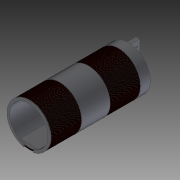
# Autodesk Inventor part: 3113_Rx Coil_V1
Saved by Autodesk Inventor 2020 (Build 240168000, 168)
## iProperties
Created: 2017-07-27
Part Number: 3113_Rx Coil_V1
Material: Acetal Resin, White
Document SubType Name: Modeling
Designer: RFLab
Density: 1.425 g/cm^3
Appearance: Smooth - White
Mass: 82.1964 g
Surface Area: 486.741 cm^2
Volume: 57.6817 cm^3
Author: RFLab
Autodesk Inventor part; units mm, degrees
ref_plane "XZ Plane" through (0, 0, 0) normal (0, 1, 0) x (-1, 0, 0)
ref_plane "XY Plane" through (0, 0, 0) normal (0, 0, 1) x (1, 0, 0)
sketch "Sketch1" plane through (0, 0, 0) normal (1, 0, 0) x (0, 1, 0)
  line L0 (0, 0) -> (0, -63.2887) construction
  line L1 (25, 58.6865) -> (25, -71.3865)
  line L2 (25, -71.3865) -> (28.75, -71.3865)
  line L3 (28.75, -71.3865) -> (28.75, -58.6865)
  line L4 (28.75, -58.6865) -> (26.2, -58.6865)
  line L5 (26.2, -58.6865) -> (26.2, -18.6865)
  line L6 (26.2, -18.6865) -> (28.75, -18.6865)
  line L7 (28.75, -18.6865) -> (28.75, 18.6865)
  line L8 (28.75, 18.6865) -> (26.2, 18.6865)
  line L9 (26.2, 18.6865) -> (26.2, 58.6865)
  line L10 (28.75, 58.6865) -> (25, 58.6865)
  line L11 (26.2, 58.6865) -> (26.2, 58.6865)
  point P0 (28.75, 0)
  dimension "d35" = 25
  dimension "d43" = 12.7
  dimension "d61" = 117.373
  dimension "d62" = 40
  dimension "d63" = 40
  dimension "d64" = 37.373
  dimension "d125" = 1.2
  dimension "d127" = 28.75
  dimension "d128" = 2.55
  constraints: 24 end point, 6 perpendicular, 6 point on line, 3 vertical, 1 collinear, 1 horizontal alignment, 1 midpoint
  measures "d35" distance between parallel lines of L0 L1
  measures "d43" distance of L2.end L3.end
  measures "d61" distance between parallel lines of L4 L10
  measures "d62" distance of L8.end L9.end
  measures "d63" distance of L4.end L5.end
  measures "d64" distance of L6.end L7.end
  measures "d125" distance between parallel lines of L1 L5
  measures "d127" distance between parallel lines of L7 L0
  measures "d128" distance between parallel lines of L5 L3
revolve "Revolution1" add sketch "Sketch1" angle 360 about axis through (0, 0, 0) along (0, 0, -1)
sketch "Sketch2" plane through (0, 0, -71.3865) normal (0, 0, -1) x (-1, 0, 0)
  line L0 (-16.1894, -19.05) -> (-11.1252, -19.05)
  line L1 (-11.1252, -19.05) -> (-11.1252, -23.8252)
  line L2 (-11.1252, -23.8252) -> (-6.35, -23.8252)
  line L3 (-6.35, -23.8252) -> (-6.35, -19.05)
  line L4 (-6.35, -19.05) -> (6.35, -19.05)
  line L5 (6.35, -19.05) -> (6.35, -23.8252)
  line L6 (6.35, -23.8252) -> (11.1252, -23.8252)
  line L7 (11.1252, -23.8252) -> (11.1252, -19.05)
  line L8 (11.1252, -19.05) -> (16.1894, -19.05)
  circle A0 centre (0, 0) radius 25 projected
  arc A1 (-16.1894, -19.05) -> (16.1894, -19.05) centre (0, 0) ccw
  point P0 (0, -19.05)
  dimension "d11" = 19.05
  dimension "d12" = 4.7752
  dimension "d14" = 12.7
  constraints: 18 end point, 6 point on line, 5 perpendicular, 2 equal length, 2 point on circle, 1 centre point, 1 coincident, 1 horizontal, 1 midpoint, 1 vertical alignment, 2 other
  measures "d11" distance from line of L4 point (0, 0)
  measures "d12" distance of L2.end L3.end
  measures "d14" distance of L3.end L4.end
extrude "Extrusion1" [suppressed]
sketch "Sketch4" plane through (0, 0, 0) normal (1, 0, 0) x (0, 1, 0)
  circle A0 centre (26.7715, -19.258) radius 0.5715
  line L0 (-28.75, -18.6865) -> (28.75, -18.6865) projected
  line L1 (26.2, -18.6865) -> (26.2, -58.6865) projected
  point P0 (0, 0)
  point P1 (26.2, -176.784)
  dimension "d22" = 1.143
  constraints: 2 point on line, 1 centre point, 1 tangent, 1 vertical alignment, 3 other
  measures "d22" diameter of A0
sketch "Sketch10" plane through (0, 0, 58.6865) normal (0, 0, 1) x (1, 0, 0)
  circle A0 centre (0, 0) radius 25 projected
  line L0 (-12.193, -21.825) -> (12.193, -21.825)
  line L1 (0, -21.825) -> (0, -25)
  dimension "d45" = 3.175
  constraints: 4 end point, 3 point on circle, 1 horizontal, 1 midpoint, 1 vertical
  measures "d45" distance of L1.start L1.end
extrude "Extrusion5" add sketch "Sketch10" against normal up to surface (130.073 mm away) contours L0 L1 A0 | A0 L1 L0
sketch "Sketch11" plane through (0, 0, 58.6865) normal (0, 0, 1) x (1, 0, 0)
  arc A0 (12.193, -21.825) -> (-12.193, -21.825) centre (0, 0) ccw projected
  line L0 (12.193, -21.825) -> (-12.2967, -21.825)
  line L1 (-12.2967, -21.825) -> (-12.2967, -41.275)
  line L2 (-12.2967, -41.275) -> (12.193, -41.275)
  line L3 (12.193, -41.275) -> (12.193, -21.825)
  line L4 (-6.35, -41.275) -> (6.35, -41.275)
  line L5 (6.35, -41.275) -> (6.35, -21.825)
  line L6 (6.35, -21.825) -> (-6.35, -21.825)
  line L7 (-6.35, -21.825) -> (-6.35, -41.275)
  arc A1 (0, 28.75) -> (0, 28.75) centre (0, 0) ccw projected
  point P0 (0, -41.275)
  point P1 (0, 28.75)
  dimension "d48" = 41.275
  dimension "d49" = 12.7
  constraints: 16 end point, 4 parallel, 2 horizontal, 2 perpendicular, 2 point on line, 1 midpoint, 1 point on circle, 1 vertical alignment
  measures "d48" distance from line of A0.centre L2
  measures "d49" distance between parallel lines of L5 L7
extrude "Extrusion6" add sketch "Sketch11" along normal blind 14 contours L5 A1 L7 L0 | L5 L2 L7 A1
sketch "Sketch12" plane through (0, 0, 72.6865) normal (0, 0, 1) x (1, 0, 0)
  line L0 (6.35, -21.825) -> (-6.35, -21.825) projected
  line L1 (0, -21.825) -> (0, -31.496)
  circle A0 centre (0, -31.496) radius 2.54
  point P0 (0, 0)
  dimension "d52" = 9.671
  dimension "d53" = 5.08
  constraints: 2 coincident, 2 end point, 1 centre point, 1 midpoint, 1 vertical
  measures "d52" distance of L1.start L1.end
  measures "d53" diameter of A0
extrude "Extrusion7" cut sketch "Sketch12" against normal blind 9.525
sketch "Sketch13" plane through (0, 0, 58.6865) normal (0, 0, -1) x (-1, 0, 0)
  arc A0 (-6.35, -27.8605) -> (6.35, -27.8605) centre (0, 0) ccw projected
  line L0 (-6.35, -41.275) -> (-6.35, -25.4188) projected
  line L1 (6.35, -41.275) -> (-6.35, -41.275) projected
  line L2 (6.35, -25.4188) -> (6.35, -41.275) projected
extrude "Extrusion8" cut sketch "Sketch13" against normal blind 8
sketch "Sketch20" plane through (0, 0, 58.6865) normal (0, 0, 1) x (1, 0, 0)
  circle A0 centre (0, 0) radius 28.58
  circle A1 centre (0, 0) radius 25
  dimension "d110" = 57.16
  dimension "d120" = 50
  constraints: 2 centre point, 2 coincident
  measures "d110" diameter of A0
  measures "d120" diameter of A1
extrude "Extrusion14" add sketch "Sketch20" along normal blind 1
ref_plane "Work Plane4" through (-30, 0, 0) normal (1, 0, 0) x (0, 1, 0)
sketch "Sketch29" plane through (-30, 0, 0) normal (1, 0, 0) x (0, 1, 0)
  line L0 (-26.2, 58.6865) -> (26.2, 58.6865) projected
  line L1 (0, 58.6865) -> (0, -71.4375)
  line L2 (-28.75, -71.3865) -> (28.75, -71.3865) projected
  line L3 (2.5, 58.6865) -> (0.5, 58.6865)
  line L4 (0.5, 58.6865) -> (0.5, -71.3865)
  line L5 (0.5, -71.3865) -> (2.5, -71.3865)
  line L6 (2.5, -71.3865) -> (2.5, 58.6865)
  line L7 (-0.5, 58.6865) -> (-2.5, 58.6865)
  line L8 (-2.5, 58.6865) -> (-2.5, -71.3865)
  line L9 (-2.5, -71.3865) -> (-0.5, -71.3865)
  line L10 (-0.5, -71.3865) -> (-0.5, 58.6865)
  point P0 (0, 0)
  dimension "d210" = 2
  dimension "d211" = 0.5
  dimension "d212" = 2
  dimension "d213" = 0.5
  constraints: 18 end point, 4 parallel, 4 point on line, 2 horizontal, 2 perpendicular, 1 midpoint, 1 vertical
  measures "d210" distance between parallel lines of L4 L6
  measures "d211" distance between parallel lines of L4 L1
  measures "d212" distance between parallel lines of L8 L10
  measures "d213" distance between parallel lines of L1 L10
extrude "Extrusion21" cut sketch "Sketch29" along normal up to surface contours L0 L10 L2 L8 | L0 L6 L2 L4 round surface about axis through (0, 0, 38.6865) along (0, 0, -1) radius 26.2 far side no
sketch "Sketch30" plane through (-26, -0.5, -71.3865) normal (0, 0, -1) x (-1, 0, 0)
  arc A0 (-13.807, -21.325) -> (-38.193, -21.325) centre (-26, 0.5) ccw projected
  line L0 (-10.9532, 20.4649) -> (-10.9532, -19.4649)
  arc A1 (-10.9532, -19.4649) -> (-10.9532, 20.4649) centre (-26, 0.5) ccw
  constraints: 4 point on circle, 2 end point, 1 centre point, 1 coincident, 1 vertical
extrude "Extrusion22" add sketch "Sketch30" against normal blind 3
sketch "Sketch31" plane through (-26, -0.5, -71.3865) normal (0, 0, -1) x (-1, 0, 0)
  line L0 (-10.9532, -19.4649) -> (-10.9532, 20.4649) projected
  line L1 (-10.9532, 10.7931) -> (-5.9532, 10.7931)
  line L2 (-5.9532, 10.7931) -> (-5.9532, -9.7931)
  line L3 (-5.9532, -9.7931) -> (-10.9532, -9.7931)
  line L4 (-10.9532, -9.7931) -> (-10.9532, 10.7931)
  point P0 (-26, 0.5)
  dimension "d219" = 9.6718
  dimension "d220" = 9.6718
  dimension "d221" = 5
  constraints: 8 end point, 2 parallel, 1 horizontal, 1 perpendicular, 1 point on line
  measures "d219" vertical distance of L0.end L1.end
  measures "d220" distance of L0.start L3.end
  measures "d221" distance of L2.end L3.end
extrude "Extrusion23" add sketch "Sketch31" along normal blind 30
sketch "Sketch32" plane through (-30, 0, 0) normal (1, 0, 0) x (0, 1, 0)
  line L0 (-2.5, -71.3865) -> (-0.5, -71.3865) projected
  circle A0 centre (-1.5, -71.3865) radius 1
  circle A1 centre (1.5875, -71.3865) radius 1
  circle A2 centre (3.2931, -77.0857) radius 1.5
  circle A3 centre (-3.2931, -77.0857) radius 1.5
  circle A4 centre (-3.2931, -85.725) radius 1.5
  circle A5 centre (3.2931, -85.725) radius 1.5
  line L1 (10.2931, -71.3865) -> (10.2931, -101.3865) projected
  line L2 (-10.2931, -71.3865) -> (-10.2931, -101.3865) projected
  line L3 (-3.7931, -94.925) -> (-2.2931, -94.925)
  line L4 (-2.2931, -94.925) -> (-2.2931, -98.425)
  line L5 (-2.2931, -98.425) -> (-3.7931, -98.425)
  line L6 (-3.7931, -98.425) -> (-3.7931, -94.925)
  line L7 (2.2931, -94.925) -> (3.7931, -94.925)
  line L8 (3.7931, -94.925) -> (3.7931, -98.425)
  line L9 (3.7931, -98.425) -> (2.2931, -98.425)
  line L10 (2.2931, -98.425) -> (2.2931, -94.925)
  point P0 (0, 0)
  dimension "d224" = 2
  dimension "d225" = 2
  dimension "d226" = 3
  dimension "d227" = 3
  dimension "d228" = 3
  dimension "d229" = 3
  dimension "d230" = 7
  dimension "d231" = 7
  dimension "d232" = 7
  dimension "d233" = 7
  dimension "d234" = 1.5
  dimension "d235" = 1.5
  dimension "d236" = 3.5
  dimension "d237" = 3.5
  dimension "d238" = 0
  dimension "d239" = 6.5
  dimension "d240" = 6.5
  dimension "d241" = 4.5861
  constraints: 16 end point, 6 centre point, 4 parallel, 2 horizontal, 2 perpendicular, 1 midpoint
  measures "d224" diameter of A0
  measures "d225" diameter of A1
  measures "d226" diameter of A2
  measures "d227" diameter of A3
  measures "d228" diameter of A4
  measures "d229" diameter of A5
  measures "d230" distance from line of L1 A2.centre
  measures "d231" distance from line of L2 A3.centre
  measures "d232" distance from line of L2 A4.centre
  measures "d233" distance from line of L1 A5.centre
  measures "d234" distance of L4.end L5.end
  measures "d235" distance of L8.end L9.end
  measures "d236" distance of L7.end L8.end
  measures "d237" distance of L3.end L4.end
  measures "d238" distance between parallel lines of L9 L5
  measures "d239" distance between parallel lines of L2 L6
  measures "d240" distance between parallel lines of L1 L8
  measures "d241" distance between parallel lines of L10 L4
extrude "Extrusion24" cut sketch "Sketch32" along normal blind 30
ref_plane "Work Plane5" through (-28.6411, 2.5, 18.6865) normal (1, 0, 0) x (0, 1, 0)
sketch "Sketch33" plane through (-28.6411, 2.5, 18.6865) normal (1, 0, 0) x (0, 1, 0)
  line L0 (-5, -37.373) -> (-4.3, -37.373)
  line L1 (-4.3, -37.373) -> (-4.3, -35.373)
  line L2 (-4.3, -35.373) -> (-5, -35.373)
  line L3 (-5, -35.373) -> (-5, -37.373)
  line L4 (0, -37.373) -> (-0.7, -37.373)
  line L5 (-0.7, -37.373) -> (-0.7, -35.373)
  line L6 (-0.7, -35.373) -> (0, -35.373)
  line L7 (0, -35.373) -> (0, -37.373)
  line L8 (-5, 0) -> (-5, -37.373) projected
  line L9 (-5, 0) -> (-4.3, 0)
  line L10 (-4.3, 0) -> (-4.3, -2)
  line L11 (-4.3, -2) -> (-5, -2)
  line L12 (-5, -2) -> (-5, 0)
  line L13 (0, 0) -> (-0.7, 0)
  line L14 (-0.7, 0) -> (-0.7, -2)
  line L15 (-0.7, -2) -> (0, -2)
  line L16 (0, -2) -> (0, 0)
  line L17 (-5, 0) -> (-5, -90.073) projected
  line L18 (-5, -77.3163) -> (-4.3, -77.3163)
  line L19 (-4.3, -77.3163) -> (-4.3, -79.3163)
  line L20 (-4.3, -79.3163) -> (-5, -79.3163)
  line L21 (-5, -79.3163) -> (-5, -77.3163)
  line L22 (0, -77.3163) -> (-0.7, -77.3163)
  line L23 (-0.7, -77.3163) -> (-0.7, -79.3163)
  line L24 (-0.7, -79.3163) -> (0, -79.3163)
  line L25 (0, -79.3163) -> (0, -77.3163)
  line L26 (0, -37.373) -> (0, 0) projected
  point P0 (-2.5, -18.6865)
  point P1 (-5, 40)
  dimension "d244" = 0.7
  dimension "d245" = 2
  dimension "d246" = 0.7
  dimension "d247" = 2
  dimension "d248" = 0
  dimension "d249" = 0.7
  dimension "d250" = 2
  dimension "d251" = 2
  dimension "d252" = 0.7
  dimension "d253" = 2
  dimension "d254" = 0.7
  dimension "d255" = 0.7
  dimension "d256" = 2
  constraints: 48 end point, 12 parallel, 6 horizontal, 6 perpendicular, 6 point on line
  measures "d244" distance of L1.end L2.end
  measures "d245" distance of L0.end L1.end
  measures "d246" distance of L4.start L4.end
  measures "d247" distance of L4.end L5.end
  measures "d248" distance from line of L26 L4.start
  measures "d249" distance of L18.start L18.end
  measures "d250" distance of L18.end L19.end
  measures "d251" distance of L22.end L23.end
  measures "d252" distance of L22.start L22.end
  measures "d253" distance of L9.end L10.end
  measures "d254" distance of L10.end L11.end
  measures "d255" distance of L14.end L15.end
  measures "d256" distance of L13.end L14.end
extrude "Extrusion25" add sketch "Sketch33" along normal blind 0.8
sketch "Sketch34" plane through (-12.193, -21.825, -71.3865) normal (0, 1, 0) x (1, 0, 0)
  line L0 (18.543, -144.073) -> (5.843, -144.073) projected
  line L1 (5.843, -130.073) -> (5.843, -144.073) projected
  line L2 (5.843, -130.073) -> (18.543, -130.073)
  line L3 (18.543, -130.073) -> (18.543, -144.073)
  line L4 (18.543, -144.073) -> (5.843, -144.073)
  line L5 (5.843, -144.073) -> (5.843, -130.073)
  point P0 (12.193, -71.3865)
  constraints: 8 end point, 2 parallel, 1 horizontal, 1 perpendicular
extrude "Extrusion26" cut sketch "Sketch34" against normal through all
sketch "Sketch35" plane through (0, 0, 0) normal (1, 0, 0) x (0, 1, 0)
  line L0 (26.2, 58.6865) -> (26.2, -58.6865) projected
  circle A0 centre (26.805, -58.0815) radius 0.605
  line L1 (2.5, -58.6865) -> (-2.5, -58.6865) projected
  line L2 (2.5, -58.6865) -> (-2.5, -58.6865) projected
  line L3 (-28.75, -58.6865) -> (28.75, -58.6865) projected
  circle A1 centre (28.015, -58.0815) radius 0.605
  line L4 (0, 106.9806) -> (0, -224.0781) projected
  point P0 (0, 0)
  point P1 (-2.5, -58.6865)
  point P2 (2.5, -58.6865)
  point P3 (27.41, -58.0815)
  dimension "d261" = 1.21
  dimension "d262" = 1.21
  constraints: 2 centre point, 1 equal radius, 1 tangent, 3 other
  measures "d261" diameter of A0
  measures "d262" diameter of A1
revolve "Revolution2" add sketch "Sketch35" angle 360 about axis through (0, 0, -6.35) along (0, 0, -1) separate body contours A0 | A1
pattern_linear "Rectangular Pattern1" count 33 spacing 1.21 along (0, 0, 1) of "Revolution2" bodies 2
pattern_linear "Rectangular Pattern2" count 2 spacing 77.37 along (0, 0, 1) of "Revolution2", "Rectangular Pattern1" bodies 2
body "Solid1"
body "Solid3"
